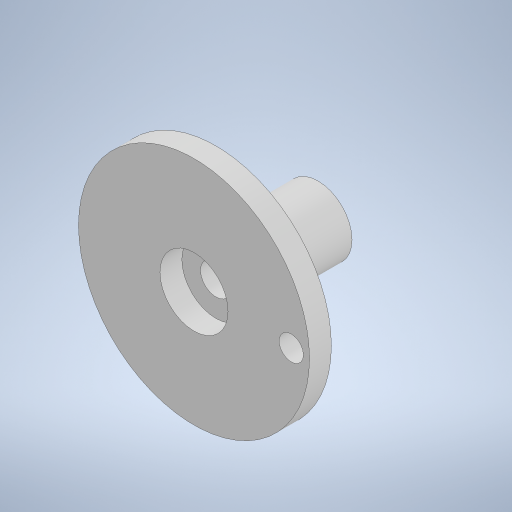
# Autodesk Inventor part: TA 212 project part(DISK)
Saved by Autodesk Inventor 2024 (Build 280153000, 153)
## iProperties
Created: 2023-08-27
Part Number: TA 212 project part(DISK)
Material: Generic
Document SubType Name: Modeling
Designer: 91865
Density: 1 g/cm^3
Appearance: Default
Author: 91865
Autodesk Inventor part; units mm, degrees
ref_plane "YZ Plane" through (0, 0, 0) normal (1, 0, 0) x (0, 1, 0)
ref_plane "XZ Plane" through (0, 0, 0) normal (0, 1, 0) x (-1, 0, 0)
ref_plane "XY Plane" through (0, 0, 0) normal (0, 0, 1) x (1, 0, 0)
sketch "Sketch1" plane through (0, 0, 0) normal (0, 0, 1) x (1, 0, 0)
  circle A0 centre (0, 0) radius 6.35
  circle A1 centre (0, 0) radius 14
  circle A2 centre (0, 0) radius 47.5
  dimension "d0" = 12.7
  dimension "d1" = 28
  dimension "d2" = 95
  constraints: 3 centre point, 3 coincident
  measures "d0" diameter of A0
  measures "d1" diameter of A1
  measures "d2" diameter of A2
extrude "Extrusion1" add sketch "Sketch1" along normal blind 9 contours A2
sketch "Sketch2" plane through (0, 0, 0) normal (0, 0, -1) x (-1, 0, 0)
  circle A0 centre (0, 0) radius 14
  circle A1 centre (0, 0) radius 6.35
  dimension "d5" = 28
  dimension "d6" = 12.7
  constraints: 2 centre point, 2 coincident
  measures "d5" diameter of A0
  measures "d6" diameter of A1
extrude "Extrusion2" add sketch "Sketch2" along normal blind 42
sketch "Sketch3" plane through (0, 0, 0) normal (0, 0, -1) x (-1, 0, 0)
  circle A0 centre (0, 0) radius 35
  arc A1 (34.8714, -2.9972) -> (34.8714, 2.9972) centre (35, 0) ccw
  circle A2 centre (35, 0) radius 5
  dimension "d9" = 70
  dimension "d10" = 6
  dimension "d11" = 10
  constraints: 5 point on circle, 3 centre point, 2 coincident
  measures "d9" diameter of A0
  measures "d10" diameter of A1
  measures "d11" diameter of A2
extrude "Extrusion3" cut sketch "Sketch3" along normal blind 9 contours A0 A2 | A0 A1 | A0 A2 A1 picked at (31.7184, 0.4122)
sketch "Sketch4" plane through (-35, 0, -9) normal (0, 0, -1) x (-1, 0, 0)
  point P0 (-35, 0)
sketch "Sketch5" plane through (0, 0, 9) normal (0, 0, 1) x (1, 0, 0)
  circle A0 centre (0, 0) radius 40
  circle A1 centre (40, 0) radius 3.5
  dimension "d14" = 80
  dimension "d15" = 7
  constraints: 1 centre point, 1 coincident, 1 horizontal alignment, 2 other
  measures "d15" diameter of A1
extrude "Extrusion4" cut sketch "Sketch5" against normal blind 9 contours A0 A1 | A0 A1 picked at (38.8994, -0.7916) picked at (41.039, -0.9083)
sketch "Sketch6" plane through (0, 0, 9) normal (0, 0, 1) x (1, 0, 0)
  circle A0 centre (40, 0) radius 3.5 projected
  circle A1 centre (40, 0) radius 5
  point P0 (0, 0)
  dimension "d18" = 10
  constraints: 1 centre point, 1 coincident
  measures "d18" diameter of A1
extrude "Extrusion5" cut sketch "Sketch6" against normal blind 9 contours A0 | A1
body "Solid1"
